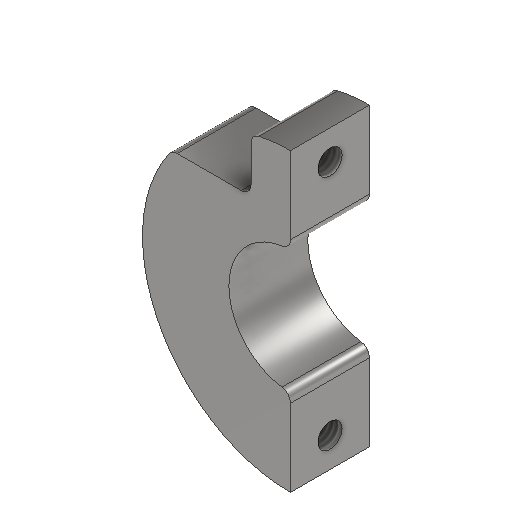
# Autodesk Inventor part: clamp-ring
Saved by Autodesk Inventor 2026.2 (Build 302298000, 298)
## iProperties
Created: 2025-10-23
Part Number: clamp-ring
Material: ステンレス鋼
Document SubType Name: Modeling
Designer: jin20
Density: 8 g/cm^3
Appearance: 半つや出し
Author: jin20
Autodesk Inventor part; units mm, degrees
ref_plane "YZ Plane" through (0, 0, 0) normal (1, 0, 0) x (0, 1, 0)
ref_plane "XZ Plane" through (0, 0, 0) normal (0, 1, 0) x (-1, 0, 0)
ref_plane "XY Plane" through (0, 0, 0) normal (0, 0, 1) x (1, 0, 0)
sketch "スケッチ1" plane through (0, 0, 0) normal (1, 0, 0) x (0, 1, 0)
  line L0 (0, 0) -> (6.25, 0) construction
  line L1 (6.25, 0) -> (6.25, 2) construction
  line L2 (6.25, 2) -> (15, 2)
  line L3 (15, 2) -> (15, 10)
  line L4 (15, 10) -> (6.25, 10)
  line L5 (6.25, 10) -> (6.25, 2)
  line L6 (0, -2) -> (0, 12) projected
  dimension "d0" = 6.25
  dimension "d4" = 8.75
  dimension "d5" = 8
  constraints: 12 end point, 2 horizontal, 2 parallel, 1 perpendicular, 1 vertical
  measures "d0" distance of L0.start L0.end
  measures "d4" distance of L4.end L3.end
  measures "d5" distance of L3.end L2.end
revolve "回転1" add sketch "スケッチ1" angle 180 about axis through (0, 0, -10) along (0, 0, 1)
sketch "スケッチ2" plane through (0, 6.25, 10) normal (0, 0, 1) x (1, 0, 0)
  line L0 (0, 8.75) -> (0, 2.75) construction
  line L1 (0, 0) -> (0, 8.75) projected
  line L2 (0, 2.75) -> (-4, 2.75) construction
  line L3 (-4, 2.75) -> (-12.5738, 2.75)
  line L4 (-12.5738, 2.75) -> (-12.5738, 9.025)
  line L5 (-12.5738, 9.025) -> (-4, 9.025)
  line L6 (-4, 9.025) -> (-4, 2.75)
  point P0 (0, -6.25)
  dimension "d7" = 6
  dimension "d8" = 4
  constraints: 12 end point, 2 parallel, 2 perpendicular, 1 horizontal, 1 point on line
  measures "d7" distance of L0.start L0.end
  measures "d8" distance of L0.end L2.end
extrude "押し出し1" cut sketch "スケッチ2" against normal through all
sketch "スケッチ4" plane through (0, -15, 2) normal (1, 0, 0) x (0, 0, -1)
  line L0 (-8, 0) -> (0, 0) projected
  line L1 (0, 0) -> (0, 8.75) projected
  point P0 (2, 15)
  point P1 (-4, 3)
  dimension "d20" = 3
  dimension "d28" = 4
  measures "d20" distance from line of L0 point (-4, 3)
  measures "d28" distance from line of L1 point (-4, 3)
hole "穴2" at (0, -12, 6) direction (-1, 0, 0) diameter 2.459 end through all thread size "M3x0.5" class "6H" standard "ANSI Metric M Profile"
fillet "フィレット2" radius 1 5 edges at (-4, 14.4568, 6) (-4, 9, 6) (-12, 9, 6) (0, 6.25, 6) (0, -6.25, 6)
sketch "スケッチ6" plane through (-4, 10, 10) normal (-1, 0, 0) x (0, 0, 1)
  line L0 (-8, 0) -> (-8, 3.6748) projected
  line L1 (-8, -1) -> (0, -1) projected
  point P0 (-10, -10)
  point P1 (-4, 2)
  dimension "d40" = 4
  dimension "d41" = 3
  measures "d40" distance from line of L0 point (-4, 2)
  measures "d41" distance from line of L1 point (-4, 2)
hole "穴4" at (-4, 12, 6) direction (1, 0, 0) diameter 2.459 end through all thread size "M3x0.5" class "6H" standard "ANSI Metric M Profile"
